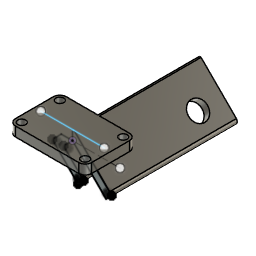
Suporte+Pi+Camera_Poncha (Autodesk Fusion 360 design; units mm, degrees)
Autodesk Fusion 360 part; units mm, degrees
note: some values were not read from the file. Set by a fixed rule: which sketch regions a step uses.
sketch "Esboço1" plane through (0, 0, 0) normal (0, 0, 1) x (1, 0, 0)
  line L0 (-10, 6) -> (10, 6)
  line L1 (10, 6) -> (10, -6)
  line L2 (10, -6) -> (-10, -6)
  line L3 (-10, -6) -> (-10, 6)
  line L4 (-10, 6) -> (10, -6) construction
  line L5 (10, 6) -> (-10, -6) construction
  circle A0 centre (-10, 6) radius 1.25
  circle A1 centre (10, 6) radius 1.25
  circle A2 centre (-10, -6) radius 1.25
  circle A3 centre (10, -6) radius 1.25
  line L6 (10, -8) -> (-10, -8)
  line L7 (-12, -6) -> (-12, 6)
  line L8 (-10, 8) -> (10, 8)
  line L9 (12, 6) -> (12, -6)
  arc A4 (12, 6) -> (10, 8) centre (10, 6) ccw
  arc A5 (-10, 8) -> (-12, 6) centre (-10, 6) ccw
  arc A6 (-12, -6) -> (-10, -8) centre (-10, -6) ccw
  arc A7 (10, -8) -> (12, -6) centre (10, -6) ccw
  dimension "d1" = 20
  dimension "d2" = 12
  dimension "d3" = 2.5
  dimension "d4" = 2.5
  dimension "d5" = 2.5
  dimension "d6" = 2.5
  dimension "d8" = 2
  constraint horizontal L0
  constraint perpendicular L0 L1
  constraint parallel L0 L2
  constraint parallel L1 L3
  constraint coincident L4 origin
  constraint coincident L5 origin
  constraint coincident L0.start L3.end
  constraint coincident L0.end L1.start
  constraint coincident L2.end L3.start
  constraint coincident L1.end L2.start
  constraint tangent L8 A4
  constraint tangent L9 A4
  constraint tangent L7 A5
  constraint tangent L8 A5
  constraint equal A4 A5
  constraint tangent L6 A6
  constraint tangent L7 A6
  constraint equal A4 A6
  constraint tangent L6 A7
  constraint tangent L9 A7
  constraint equal A4 A7
  measures "d1" distance of L1.end L2.end
  measures "d2" distance of L0.end L1.end
  measures "d3" diameter of A0
  measures "d4" diameter of A1
  measures "d5" diameter of A2
  measures "d6" diameter of A3
  measures "d8" radius of A4
extrude "Extrusão1" add sketch "Esboço1" along normal blind 3 contours L0 L1 L2 L3 A0 A1 A2 A3 | L6 L7 L8 L9 A4 A5 A6 A7
sketch "Esboço2" plane through (0, 0, 0) normal (0, 1, 0) x (1, 0, 0)
  line L0 (0, 0) -> (10.6066, 10.6066)
  line L1 (0, 0) -> (15, 0) construction
  line L2 (10.6066, 10.6066) -> (11.6673, 9.5459)
  line L3 (0, 0) -> (-2.1213, 2.1213)
  line L4 (-2.1213, 3.5355) -> (2.8284, 8.4853)
  line L5 (2.8284, 9.8995) -> (2.4749, 10.253)
  line L6 (1.0607, 10.253) -> (-5.6569, 3.5355)
  line L7 (-5.6569, 2.1213) -> (-3.5355, 0)
  line L8 (-3.5355, 0) -> (0, 0)
  arc A0 (11.6673, 8.1317) -> (11.6673, 9.5459) centre (10.9602, 8.8388) ccw
  arc A1 (-5.6569, 3.5355) -> (-5.6569, 2.1213) centre (-4.9497, 2.8284) ccw
  arc A2 (-2.1213, 3.5355) -> (-2.1213, 2.1213) centre (-1.4142, 2.8284) ccw
  arc A3 (2.4749, 10.253) -> (1.0607, 10.253) centre (1.7678, 9.5459) ccw
  arc A4 (2.8284, 8.4853) -> (2.8284, 9.8995) centre (2.1213, 9.1924) ccw
  line L9 (10, -3) -> (-10, -3)
  line L10 (11.6673, 8.1317) -> (0.5355, -3)
  line L11 (0.5355, -3) -> (0, -3)
  line L12 (0, -3) -> (0, 0)
  point P0 (12.3744, 8.8388)
  point P1 (-2.8284, 2.8284)
  point P2 (3.5355, 9.1924)
  point P3 (1.7678, 10.9602)
  point P4 (-6.364, 2.8284)
  dimension "d11" = 15
  dimension "d12" = 45
  dimension "d13" = 2.5
  dimension "d14" = 4
  dimension "d15" = 9
  dimension "d16" = 2.5
  dimension "d17" = 11.5
  dimension "d18" = 4
  dimension "d19" = 1
  dimension "d28" = 2.5
  constraint horizontal L1
  constraint coincident L0.start L1.start
  constraint perpendicular L0 L2
  constraint perpendicular L0 L3
  constraint perpendicular L3 L4
  constraint perpendicular L4 L5
  constraint perpendicular L3 L6
  constraint perpendicular L6 L7
  constraint coincident P0 L2
  constraint tangent L2 A0
  constraint coincident P4 L6
  constraint coincident P4 L7
  constraint tangent L6 A1
  constraint tangent L7 A1
  constraint equal A0 A1
  constraint coincident P1 L3
  constraint coincident P1 L4
  constraint tangent L3 A2
  constraint tangent L4 A2
  constraint equal A0 A2
  constraint coincident P3 L5
  constraint coincident P3 L6
  constraint tangent L5 A3
  constraint tangent L6 A3
  constraint equal A0 A3
  constraint coincident P2 L4
  constraint coincident P2 L5
  constraint tangent L4 A4
  constraint tangent L5 A4
  constraint equal A0 A4
  constraint horizontal L9
  constraint tangent A0 L10
  constraint parallel L0 L10
  constraint coincident L9 L10.end
  constraint midpoint L9 L11.end
  constraint perpendicular L8 L12
  measures "d11" distance of L0.start L0.end
  measures "d12" angle of L0 L1
  measures "d13" distance of L0.end P0
  measures "d14" distance of L0.start P1
  measures "d15" distance of P1 P2
  measures "d16" distance of P2 P3
  measures "d17" distance of P3 P4
  measures "d18" distance of P4 L7.end
  measures "d19" radius of A0
  measures "d28" distance of L0 L10
extrude "Extrusão2" add sketch "Esboço2" along normal blind 40 contours L0 L2 A0 L9 L10 L11 L12
extrude "Extrusão3" add sketch "Esboço2" along normal blind 5 contours L3 L4 L5 L6 L7 L8 A1 A2 A3 A4
sketch "Esboço4" plane through (1.7678, 0, 1.7678) normal (0.707107, 0, 0.707107) x (0, 1, 0)
  line L0 (8, -2.5) -> (0, -2.5)
  line L1 (0, -2.5) -> (0, -14)
  line L2 (0, -14) -> (40, -14)
  line L3 (40, -14) -> (40, 1.7426)
  line L4 (40, 1.7426) -> (8, 1.7426)
  line L5 (8, 1.7426) -> (8, -2.5)
  circle A0 centre (32, -8.25) radius 3
  line L6 (0, -8.25) -> (40, -8.25)
  point P0 (0, -8.25)
  dimension "d29" = 6
  dimension "d30" = 32
  constraint midpoint L1 P0
  constraint coincident P0 L6.start
  constraint coincident L3 L6.end
  constraint perpendicular L3 L6
  constraint coincident A0.centre L6
  measures "d29" diameter of A0
  measures "d30" distance of P0 A0.centre
extrude "Extrusão5" cut sketch "Esboço4" against normal blind 2.5 contours A0 L6 | A0 L6
equation "d4 = d3"
equation "d5 = d3"
equation "d6 = d3"
equation "d17 = 9 mm + 2.5 mm"
equation "d20 = 20 mm + 20 mm"
equation "d30 = d20 - 8 mm"
named bodies: "Suporte_RPi_Poncha"
